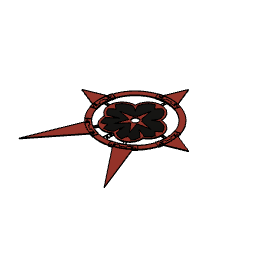
ワカモ_ヘイロー_mk1 v11 (Autodesk Fusion 360 design; units mm, degrees)
Autodesk Fusion 360 part; units mm, degrees
sketch "スケッチ1" plane through (0, 0, 0) normal (0, 0, 1) x (1, 0, 0) in component "main"
  circle A0 centre (0, 0) radius 95
  circle A1 centre (0, 0) radius 10
  line L0 (0, 0) -> (0, 47.5) construction
  line L1 (0, 0) -> (47.5, 0) construction
  line L2 (0, 0) -> (-47.5, 0) construction
  line L3 (0, 0) -> (23.75, -41.1362) construction
  line L4 (0, 0) -> (-23.75, -41.1362) construction
  line L5 (0, 47.5) -> (-6.6163, 13.462)
  line L6 (0, 47.5) -> (6.6163, 13.462)
  line L7 (-47.5, 0) -> (-13.462, 6.6163)
  line L8 (-47.5, 0) -> (-13.462, -6.6163)
  line L9 (-23.75, -41.1362) -> (-12.4609, -8.3502)
  line L10 (-23.75, -41.1362) -> (-1.0011, -14.9666)
  line L11 (23.75, -41.1362) -> (1.0011, -14.9666)
  line L12 (23.75, -41.1362) -> (12.4609, -8.3502)
  line L13 (47.5, 0) -> (13.462, -6.6163)
  line L14 (47.5, 0) -> (13.462, 6.6163)
  arc A2 (-13.462, -6.6163) -> (-12.4609, -8.3502) centre (0, 0) ccw
  arc A3 (-1.0011, -14.9666) -> (1.0011, -14.9666) centre (0, 0) ccw
  arc A4 (12.4609, -8.3502) -> (13.462, -6.6163) centre (0, 0) ccw
  arc A5 (13.462, 6.6163) -> (6.6163, 13.462) centre (0, 0) ccw
  arc A6 (-6.6163, 13.462) -> (-13.462, 6.6163) centre (0, 0) ccw
  circle A7 centre (0, 40) radius 40 construction
  circle A8 centre (40, 0) radius 40 construction
  circle A9 centre (-40, 0) radius 40 construction
  circle A10 centre (-23.75, -41.1362) radius 35 construction
  circle A11 centre (23.75, -41.1362) radius 35 construction
  arc A12 (40, 40) -> (-40, 40) centre (0, 40) ccw
  arc A13 (58.304, -35.5663) -> (40, 40) centre (40, 0) ccw
  arc A14 (-40, 40) -> (-58.304, -35.5663) centre (-40, 0) ccw
  arc A15 (0, -66.8449) -> (58.304, -35.5663) centre (23.75, -41.1362) ccw
  arc A16 (-58.304, -35.5663) -> (0, -66.8449) centre (-23.75, -41.1362) ccw
  circle A17 centre (0, 40) radius 34 construction
  circle A18 centre (-40, 0) radius 34 construction
  circle A19 centre (40, 0) radius 34 construction
  circle A20 centre (-23.75, -41.1362) radius 29 construction
  circle A21 centre (23.75, -41.1362) radius 29 construction
  line L15 (0, 40) -> (0, 59.4286) construction
  line L16 (0, 59.4286) -> (-10.7604, 72.2523)
  line L17 (0, 59.4286) -> (10.7604, 72.2523)
  line L18 (-40, 0) -> (-59.4286, 0) construction
  line L19 (-59.4286, 0) -> (-72.2523, 10.7604)
  line L20 (-59.4286, 0) -> (-72.2523, -10.7604)
  line L21 (40, 0) -> (59.4286, 0) construction
  line L22 (59.4286, 0) -> (72.2523, 10.7604)
  line L23 (59.4286, 0) -> (72.2523, -10.7604)
  line L24 (-23.75, -41.1362) -> (-31, -53.6936) construction
  line L25 (-31, -53.6936) -> (-28.1602, -69.7989)
  line L26 (-31, -53.6936) -> (-46.3675, -59.2869)
  line L27 (23.75, -41.1362) -> (31, -53.6936) construction
  line L28 (31, -53.6936) -> (28.1602, -69.7989)
  line L29 (31, -53.6936) -> (46.3675, -59.2869)
  arc A22 (33.997, 39.547) -> (10.7604, 72.2523) centre (0, 40) ccw
  arc A23 (-10.7604, 72.2523) -> (-33.997, 39.547) centre (0, 40) ccw
  arc A24 (-39.547, 33.997) -> (-72.2523, 10.7604) centre (-40, 0) ccw
  arc A25 (-72.2523, -10.7604) -> (-56.7833, -29.5689) centre (-40, 0) ccw
  arc A26 (-52.5768, -37.9714) -> (-46.3675, -59.2869) centre (-23.75, -41.1362) ccw
  arc A27 (-28.1602, -69.7989) -> (-4.0421, -62.4106) centre (-23.75, -41.1362) ccw
  arc A28 (4.0421, -62.4106) -> (28.1602, -69.7989) centre (23.75, -41.1362) ccw
  arc A29 (46.3675, -59.2869) -> (52.5768, -37.9714) centre (23.75, -41.1362) ccw
  arc A30 (56.7833, -29.5689) -> (72.2523, -10.7604) centre (40, 0) ccw
  arc A31 (72.2523, 10.7604) -> (39.547, 33.997) centre (40, 0) ccw
  line L30 (0, 0) -> (-33.3417, 33.3417) construction
  circle A32 centre (0, 0) radius 35 construction
  line L31 (-39.547, 33.997) -> (-24.7487, 24.7487)
  line L32 (-33.997, 39.547) -> (-24.7487, 24.7487)
  line L33 (0, 0) -> (33.3417, 33.3417) construction
  line L34 (33.997, 39.547) -> (24.7487, 24.7487)
  line L35 (39.547, 33.997) -> (24.7487, 24.7487)
  line L36 (0, 0) -> (-51.296, -32.0687) construction
  line L37 (-56.7833, -29.5689) -> (-29.6777, -18.5536)
  line L38 (-29.6777, -18.5536) -> (-52.5768, -37.9714)
  line L39 (0, 0) -> (0, -57.7776) construction
  line L40 (-4.0421, -62.4106) -> (0, -35)
  line L41 (0, -35) -> (4.0421, -62.4106)
  line L42 (0, 0) -> (51.296, -32.0687) construction
  line L43 (52.5768, -37.9714) -> (29.6777, -18.5536)
  line L44 (56.7833, -29.5689) -> (29.6777, -18.5536)
  line L45 (-2.5, 79.9218) -> (-2.5, 94.9671)
  line L46 (2.5, 79.9218) -> (2.5, 94.9671)
  line L47 (-94.9671, 2.5) -> (-79.9218, 2.5)
  line L48 (-94.9671, -2.5) -> (-79.9218, -2.5)
  line L49 (79.9218, 2.5) -> (94.9671, 2.5)
  line L50 (79.9218, -2.5) -> (94.9671, -2.5)
  line L51 (38.5875, -72.8355) -> (44.8782, -83.7314)
  line L52 (43.7837, -69.8355) -> (50.0744, -80.7314)
  line L53 (-43.7837, -69.8355) -> (-50.0744, -80.7314)
  line L54 (-38.5875, -72.8355) -> (-44.8782, -83.7314)
  circle A33 centre (-42.75, -74.0452) radius 1.6
  circle A34 centre (42.75, -74.0452) radius 1.6
  line L55 (-73.3227, -81.9987) -> (-34.3516, -104.4987) construction
  line L56 (-53.8371, -93.2487) -> (-31, -53.6936) construction
  line L57 (-71.3227, -78.5346) -> (-70.094, -77.6742)
  line L58 (-70.094, -77.6742) -> (-69.094, -75.9421)
  line L59 (-69.094, -75.9421) -> (-68.9632, -74.4479)
  line L60 (-73.3227, -81.9987) -> (-71.3227, -78.5346)
  line L61 (-68.9632, -74.4479) -> (-68.2035, -73.1319)
  line L62 (-56.7679, -82.325) -> (-58.7679, -85.7891)
  arc A35 (-68.2035, -73.1319) -> (-56.7679, -82.325) centre (0, 0) ccw
  line L63 (-58.7679, -85.7891) -> (-51.8397, -89.7891)
  arc A36 (-42.9115, -90.325) -> (-29.2324, -95.6319) centre (0, 0) ccw
  line L64 (-29.9921, -96.9479) -> (-29.2324, -95.6319)
  line L65 (-31.2208, -97.8082) -> (-29.9921, -96.9479)
  line L66 (-32.2208, -99.5403) -> (-31.2208, -97.8082)
  line L67 (-32.3516, -101.0346) -> (-32.2208, -99.5403)
  line L68 (-34.3516, -104.4987) -> (-32.3516, -101.0346)
  line L69 (-42.9115, -90.325) -> (-44.9115, -93.7891)
  line L70 (-44.9115, -93.7891) -> (-51.8397, -89.7891)
  line L71 (-69.594, -76.8082) -> (-73.9241, -74.3082) construction
  circle A37 centre (-73.9241, -74.3082) radius 1.5
  circle A38 centre (-27.3907, -101.1742) radius 1.5
  circle A39 centre (27.3907, -101.1742) radius 1.5
  line L72 (31.2208, -97.8082) -> (29.9921, -96.9479)
  line L73 (29.9921, -96.9479) -> (29.2324, -95.6319)
  arc A40 (29.2324, -95.6319) -> (42.9115, -90.325) centre (0, 0) ccw
  line L74 (32.2208, -99.5403) -> (31.2208, -97.8082)
  line L75 (32.3516, -101.0346) -> (32.2208, -99.5403)
  line L76 (34.3516, -104.4987) -> (32.3516, -101.0346)
  line L77 (42.9115, -90.325) -> (44.9115, -93.7891)
  line L78 (44.9115, -93.7891) -> (51.8397, -89.7891)
  line L79 (58.7679, -85.7891) -> (51.8397, -89.7891)
  line L80 (56.7679, -82.325) -> (58.7679, -85.7891)
  arc A41 (56.7679, -82.325) -> (68.2035, -73.1319) centre (0, 0) ccw
  line L81 (68.9632, -74.4479) -> (68.2035, -73.1319)
  line L82 (69.094, -75.9421) -> (68.9632, -74.4479)
  line L83 (70.094, -77.6742) -> (69.094, -75.9421)
  line L84 (71.3227, -78.5346) -> (70.094, -77.6742)
  line L85 (73.3227, -81.9987) -> (71.3227, -78.5346)
  circle A42 centre (73.9241, -74.3082) radius 1.5
  circle A43 centre (101.3148, -26.8661) radius 1.5
  line L86 (100.3148, -21.8661) -> (98.9554, -22.5)
  line L87 (98.9554, -22.5) -> (97.4359, -22.5)
  arc A44 (97.4359, -22.5) -> (99.6795, -8) centre (0, 0) ccw
  line L88 (102.3148, -21.8661) -> (100.3148, -21.8661)
  line L89 (103.6743, -22.5) -> (102.3148, -21.8661)
  line L90 (107.6743, -22.5) -> (103.6743, -22.5)
  line L91 (99.6795, -8) -> (103.6795, -8)
  line L92 (103.6795, -8) -> (103.6795, 0)
  line L93 (103.6795, 8) -> (103.6795, 0)
  line L94 (99.6795, 8) -> (103.6795, 8)
  arc A45 (99.6795, 8) -> (97.4359, 22.5) centre (0, 0) ccw
  line L95 (98.9554, 22.5) -> (97.4359, 22.5)
  line L96 (100.3148, 21.8661) -> (98.9554, 22.5)
  line L97 (102.3148, 21.8661) -> (100.3148, 21.8661)
  line L98 (103.6743, 22.5) -> (102.3148, 21.8661)
  line L99 (107.6743, 22.5) -> (103.6743, 22.5)
  circle A46 centre (101.3148, 26.8661) radius 1.5
  circle A47 centre (26.8661, 101.3148) radius 1.5
  line L100 (21.8661, 100.3148) -> (22.5, 98.9554)
  line L101 (22.5, 98.9554) -> (22.5, 97.4359)
  arc A48 (22.5, 97.4359) -> (8, 99.6795) centre (0, 0) ccw
  line L102 (21.8661, 102.3148) -> (21.8661, 100.3148)
  line L103 (22.5, 103.6743) -> (21.8661, 102.3148)
  line L104 (22.5, 107.6743) -> (22.5, 103.6743)
  line L105 (8, 99.6795) -> (8, 103.6795)
  line L106 (8, 103.6795) -> (0, 103.6795)
  line L107 (-8, 103.6795) -> (0, 103.6795)
  line L108 (-8, 99.6795) -> (-8, 103.6795)
  arc A49 (-8, 99.6795) -> (-22.5, 97.4359) centre (0, 0) ccw
  line L109 (-22.5, 98.9554) -> (-22.5, 97.4359)
  line L110 (-21.8661, 100.3148) -> (-22.5, 98.9554)
  line L111 (-21.8661, 102.3148) -> (-21.8661, 100.3148)
  line L112 (-22.5, 103.6743) -> (-21.8661, 102.3148)
  line L113 (-22.5, 107.6743) -> (-22.5, 103.6743)
  circle A50 centre (-26.8661, 101.3148) radius 1.5
  circle A51 centre (-101.3148, 26.8661) radius 1.5
  line L114 (-100.3148, 21.8661) -> (-98.9554, 22.5)
  line L115 (-98.9554, 22.5) -> (-97.4359, 22.5)
  arc A52 (-97.4359, 22.5) -> (-99.6795, 8) centre (0, 0) ccw
  line L116 (-102.3148, 21.8661) -> (-100.3148, 21.8661)
  line L117 (-103.6743, 22.5) -> (-102.3148, 21.8661)
  line L118 (-107.6743, 22.5) -> (-103.6743, 22.5)
  line L119 (-99.6795, 8) -> (-103.6795, 8)
  line L120 (-103.6795, 8) -> (-103.6795, 0)
  line L121 (-103.6795, -8) -> (-103.6795, 0)
  line L122 (-99.6795, -8) -> (-103.6795, -8)
  arc A53 (-99.6795, -8) -> (-97.4359, -22.5) centre (0, 0) ccw
  line L123 (-98.9554, -22.5) -> (-97.4359, -22.5)
  line L124 (-100.3148, -21.8661) -> (-98.9554, -22.5)
  line L125 (-102.3148, -21.8661) -> (-100.3148, -21.8661)
  line L126 (-103.6743, -22.5) -> (-102.3148, -21.8661)
  line L127 (-107.6743, -22.5) -> (-103.6743, -22.5)
  circle A54 centre (-101.3148, -26.8661) radius 1.5
  arc A55 (-107.6743, -22.5) -> (-73.3227, -81.9987) centre (0, 0) ccw
  arc A56 (-22.5, 107.6743) -> (-107.6743, 22.5) centre (0, 0) ccw
  arc A57 (107.6743, 22.5) -> (22.5, 107.6743) centre (0, 0) ccw
  arc A58 (-34.3516, -104.4987) -> (34.3516, -104.4987) centre (0, 0) ccw
  arc A59 (73.3227, -81.9987) -> (107.6743, -22.5) centre (0, 0) ccw
  line L128 (-5, -70.6902) -> (-5, -94.8683)
  line L129 (5, -70.6902) -> (5, -94.8683)
  circle A60 centre (0, -75) radius 2.6
  circle A61 centre (0, -87) radius 2.6
  dimension "d1" = 220
  dimension "d2" = 190
  dimension "d3" = 20
  dimension "d4" = 47.5
  dimension "d5" = 47.5
  dimension "d6" = 47.5
  dimension "d7" = 60
  dimension "d8" = 47.5
  dimension "d9" = 60
  dimension "d10" = 47.5
  dimension "d11" = 30
  dimension "d12" = 11
  dimension "d13" = 11
  dimension "d14" = 11
  dimension "d15" = 11
  dimension "d16" = 11
  dimension "d17" = 11
  dimension "d18" = 11
  dimension "d19" = 11
  dimension "d20" = 11
  dimension "d21" = 11
  dimension "d22" = 40
  dimension "d23" = 40
  dimension "d24" = 40
  dimension "d25" = 80
  dimension "d26" = 80
  dimension "d27" = 80
  dimension "d28" = 70
  dimension "d29" = 70
  dimension "d30" = 68
  dimension "d31" = 68
  dimension "d32" = 68
  dimension "d33" = 58
  dimension "d34" = 58
  dimension "d35" = 19.4286
  dimension "d36" = 140
  dimension "d37" = 140
  dimension "d38" = 19.4286
  dimension "d39" = 140
  dimension "d40" = 140
  dimension "d41" = 19.4286
  dimension "d42" = 140
  dimension "d43" = 140
  dimension "d44" = 14.5
  dimension "d45" = 140
  dimension "d46" = 140
  dimension "d47" = 14.5
  dimension "d48" = 140
  dimension "d49" = 140
  dimension "d50" = 70
  dimension "d52" = 5
  dimension "d53" = 5
  dimension "d54" = 6
  dimension "d55" = 6
  dimension "d56" = 5
  dimension "d67" = 3.2
  dimension "d68" = 38
  dimension "d69" = 3
  dimension "d70" = 3.2
  dimension "d71" = 38
  dimension "d72" = 3
  dimension "d73" = 45
  dimension "d75" = 25
  dimension "d76" = 1.5
  dimension "d77" = 2
  dimension "d78" = 25
  dimension "d79" = 1.5
  dimension "d80" = 4
  dimension "d83" = 100
  dimension "d84" = 4
  dimension "d85" = 8
  dimension "d86" = 5
  dimension "d87" = 3
  dimension "d89" = 360
  dimension "d111" = 10
  dimension "d112" = 5.2
  dimension "d113" = 5.2
  dimension "d114" = 12
  dimension "d115" = 87
  constraint coincident A0.centre A1.centre
  constraint concentric A0 A58
  constraint concentric A0 A1
  constraint vertical L0
  constraint perpendicular L0 L1
  constraint perpendicular L0 L2
  constraint concentric A0 A2
  constraint coincident L5.end A2
  constraint coincident L6.end A2
  constraint coincident L10.end A2
  constraint coincident L11.end A2
  constraint coincident L12.end A2
  constraint coincident L13.end A2
  constraint coincident L14.end A2
  constraint concentric A2 A3
  constraint concentric A3 A4
  constraint concentric A4 A5
  constraint concentric A5 A6
  constraint coincident L0 A7.centre
  constraint coincident L1 A8.centre
  constraint coincident L2 A9.centre
  constraint coincident L4.end L9.start
  constraint coincident L3.end L11.start
  constraint coincident A7 A12.start
  constraint coincident A8 A12.start
  constraint coincident A9 A12.end
  constraint coincident A7 A12.end
  constraint coincident A7.centre A12.centre
  constraint coincident A11 A13.start
  constraint coincident A8.centre A13.centre
  constraint coincident A10 A14.end
  constraint coincident A9.centre A14.centre
  constraint coincident A13.start A15.end
  constraint coincident A10 A15.start
  constraint coincident A14.end A16.start
  constraint coincident A11 A15.start
  constraint concentric A7 A17
  constraint concentric A14 A18
  constraint concentric A8 A19
  constraint concentric A10 A20
  constraint concentric A11 A21
  constraint parallel L0 L15
  constraint coincident A17 L16.end
  constraint coincident A17 L17.end
  constraint parallel L2 L18
  constraint coincident A18 L19.end
  constraint coincident A18 L20.end
  constraint parallel L1 L21
  constraint coincident A19 L22.end
  constraint coincident A19 L23.end
  constraint parallel L4 L24
  constraint coincident A20 L25.end
  constraint coincident A20 L26.end
  constraint coincident A21 L28.end
  constraint coincident A21 L29.end
  constraint coincident L17.end A22.end
  constraint coincident A8 A22.start
  constraint coincident L16.end A23.start
  constraint coincident A9 A23.end
  constraint coincident L19.end A24.end
  constraint coincident A7 A24.start
  constraint coincident L20.end A25.start
  constraint coincident A10 A25.end
  constraint coincident L26.end A26.end
  constraint coincident A9 A26.start
  constraint coincident L25.end A27.start
  constraint coincident A11 A27.end
  constraint coincident L28.end A28.end
  constraint coincident A10 A28.start
  constraint coincident L29.end A29.start
  constraint coincident A8 A29.end
  constraint coincident L23.end A30.end
  constraint coincident A11 A30.start
  constraint coincident L22.end A31.start
  constraint coincident A7 A31.end
  constraint coincident A17 L30.end
  constraint coincident A18 L30.end
  constraint concentric A6 A32
  constraint coincident A32 L31.end
  constraint coincident L30 L31.end
  constraint coincident A17 L33.end
  constraint coincident A19 L33.end
  constraint coincident L33 L34.end
  constraint coincident A32 L34.end
  constraint coincident A20 L36.end
  constraint coincident A18 L36.end
  constraint coincident L36 L37.end
  constraint coincident A32 L37.end
  constraint coincident A20 L39.end
  constraint coincident A21 L39.end
  constraint coincident L39 L40.end
  constraint coincident A32 L40.end
  constraint coincident A21 L42.end
  constraint coincident A19 L42.end
  constraint coincident L42 L43.end
  constraint coincident A32 L43.end
  constraint coincident A12 L45.start
  constraint coincident A0 L45.end
  constraint vertical L45
  constraint coincident A7 L46.start
  constraint coincident A0 L46.end
  constraint parallel L45 L46
  constraint symmetric L15 L45 L46
  constraint parallel L3 L27
  constraint coincident A0 L47.start
  constraint coincident A9 L47.end
  constraint coincident A0 L48.start
  constraint coincident A14 L48.end
  constraint coincident A13 L49.start
  constraint coincident A0 L49.end
  constraint parallel L48 L49
  constraint coincident A13 L50.start
  constraint coincident A0 L50.end
  constraint parallel L49 L50
  constraint coincident A15 L51.start
  constraint coincident A0 L51.end
  constraint coincident A15 L52.start
  constraint coincident A0 L52.end
  constraint parallel L51 L52
  constraint coincident A10 L53.start
  constraint coincident A0 L53.end
  constraint coincident A16 L54.start
  constraint coincident A0 L54.end
  constraint symmetric L18 L47 L48
  constraint symmetric L24 L53 L54
  constraint symmetric L27 L51 L52
  constraint symmetric L21 L49 L50
  constraint parallel L24 L53
  constraint perpendicular L24 L55
  constraint midpoint L55 L56.start
  constraint perpendicular L55 L60
  constraint coincident L59.end L60
  constraint collinear L60 L61
  constraint parallel L53 L62
  constraint coincident L56 L63.end
  constraint perpendicular L56 L63
  constraint symmetric L55.start L56 L55.end
  constraint symmetric L56 L57.start L67.start
  constraint symmetric L56 L57.end L66.start
  constraint symmetric L56 L58.end L65.start
  constraint symmetric L56 L59.end L64.start
  constraint symmetric L56 L62.end L69.end
  constraint symmetric L56 L61.end A36.end
  constraint symmetric L56 A35 A36
  constraint symmetric L56 L62.start A36.start
  constraint symmetric L56 L63.end L70.end
  constraint coincident L55 L68.start
  constraint midpoint L58 L71.start
  constraint perpendicular L58 L71
  constraint coincident L71.end A37.centre
  constraint symmetric L56 A37 A38
  constraint concentric A55 A58
  constraint concentric A56 A58
  constraint concentric A57 A58
  constraint concentric A58 A59
  constraint coincident A10 L128.start
  constraint coincident A0 L128.end
  constraint vertical L128
  constraint coincident A11 L129.start
  constraint coincident A0 L129.end
  constraint parallel L128 L129
  constraint symmetric L39 L128 L129
  measures "d1" diameter of A58
  measures "d2" diameter of A0
  measures "d3" diameter of A1
  measures "d4" distance of A0.centre L0.end
  measures "d5" distance of A0.centre L1.end
  measures "d6" distance of A0.centre L2.end
  measures "d7" angle of L1 L3
  measures "d8" distance of A0.centre L3.end
  measures "d9" angle of L2 L4
  measures "d10" distance of A0.centre L4.end
  measures "d11" diameter of A2
  measures "d12" angle of L0 L5
  measures "d13" angle of L0 L6
  measures "d14" angle of L1 L14
  measures "d15" angle of L1 L13
  measures "d16" angle of L3 L12
  measures "d17" angle of L3 L11
  measures "d18" angle of L2 L7
  measures "d19" angle of L2 L8
  measures "d20" angle of L4 L9
  measures "d21" angle of L4 L10
  measures "d22" distance of A0.centre A7.centre
  measures "d23" distance of A0.centre A8.centre
  measures "d24" distance of A0.centre A9.centre
  measures "d25" diameter of A7
  measures "d26" diameter of A8
  measures "d27" diameter of A9
  measures "d28" diameter of A10
  measures "d29" diameter of A11
  measures "d30" diameter of A17
  measures "d31" diameter of A18
  measures "d32" diameter of A19
  measures "d33" diameter of A20
  measures "d34" diameter of A21
  measures "d35" distance of A7.centre L15.end
  measures "d36" angle of L15 L16
  measures "d37" angle of L15 L17
  measures "d38" distance of A9.centre L18.end
  measures "d39" angle of L18 L20
  measures "d40" angle of L18 L19
  measures "d41" distance of A8.centre L21.end
  measures "d42" angle of L21 L22
  measures "d43" angle of L21 L23
  measures "d44" distance of L4.end L24.end
  measures "d45" angle of L24 L26
  measures "d46" angle of L24 L25
  measures "d47" distance of L3.end L27.end
  measures "d48" angle of L27 L28
  measures "d49" angle of L27 L29
  measures "d50" diameter of A32
  measures "d52" distance of L45 L46
  measures "d53" distance of L47 L48
  measures "d54" distance of L53 L54
  measures "d55" distance of L51 L52
  measures "d56" distance of L49 L50
  measures "d67" diameter of A33
  measures "d68" distance of L4.end A33.centre
  measures "d69" distance of L54 A33.centre
  measures "d70" diameter of A34
  measures "d71" distance of L3.end A34.centre
  measures "d72" distance of L51 A34.centre
  measures "d73" distance of L55.start L55.end
  measures "d75" angle of L57 L60
  measures "d76" distance of L57.start L57.end
  measures "d77" distance of L57.end L58.end
  measures "d78" angle of L59 L60
  measures "d79" distance of L58.end L59.end
  measures "d80" distance of L55 L57.start
  measures "d83" radius of A35
  measures "d84" distance of L62.end L62.start
  measures "d85" distance of L62.end L63.end
  measures "d86" distance of L71.start L71.end
  measures "d87" diameter of A37
  measures "d111" distance of L128 L129
  measures "d112" diameter of A60
  measures "d113" diameter of A61
  measures "d114" distance of A60.centre A61.centre
  measures "d115" distance of A0.centre A61.centre
extrude "押し出し1" add sketch "スケッチ1" along normal blind 2 contours L57 L58 L59 L60 L61 L62 A35 L63 A36 L64 L65 L66 L67 L68 L69 L70 L72 L73 A40 L74 L75 L76 L77 L78 L79 L80 A41 L81 L82 L83 L84 L85 L86 L87 A44 L88 L89 L90 L91 L92 L93 L94 A45 L95 L96 L97 L98 L99 L100 L101 A48 L102 L103 L104 L105 L106 L107 L108 A49 L109 L110 L111 L112 L113 L114 L115 A52 L116 L117 L118 L119 L120 L121 L122 A53 L123 L124 L125 L126 L127 A55 A56 A57 A58 A59 makes body 1 in component "main"
extrude "押し出し2" add sketch "スケッチ1" along normal blind 2 separate body contours A0 A13 L49 L50 | A0 A12 L45 L46 | A0 A15 L51 L52 | A0 A14 L47 L48 | A0 A15 A16 L128 L129 | A0 A16 L53 L54 | A33 | A34 makes body 2 at (-45.3226, -73.8337, 0) makes body 3 at (-84.9601, -1.9446, 0) makes body 4 at (45.3226, -73.8337, 0) makes body 5 at (-1.9446, 84.9601, 0) makes body 6 at (84.9601, 1.9446, 2) makes body 7 at (-0.0648, -93.1878, 0) in component "main"
extrude "押し出し3" add sketch "スケッチ1" along normal blind 2 separate body contours A12 A13 A14 A15 A16 makes body 8 in component "main"
extrude "押し出し4" add sketch "スケッチ1" along normal blind 2 separate body contours L16 L17 L19 L20 L22 L23 L25 L26 L28 L29 A22 A23 A24 A25 A26 A27 A28 A29 A30 A31 L31 L32 L34 L35 L37 L38 L40 L41 L43 L44 makes body 9 in component "main"
extrude "押し出し5" add sketch "スケッチ1" along normal blind 2 separate body contours L5 L6 L7 L8 L9 L10 L11 L12 L13 L14 A2 A3 A4 A5 A6 makes body 10 in component "main"
sketch "スケッチ1 (2)" plane through (0, 0, 2) normal (0, 0, 1) x (-1, 0, 0) in component "突起a"
  circle A0 centre (-73.9241, 74.3082) radius 1.5
  circle A1 centre (101.3148, 26.8661) radius 1.5
  circle A2 centre (-27.3907, 101.1742) radius 1.5
  circle A3 centre (-26.8661, -101.3148) radius 1.5
  circle A4 centre (27.3907, 101.1742) radius 1.5
  circle A5 centre (101.3148, -26.8661) radius 1.5
  circle A6 centre (-101.3148, 26.8661) radius 1.5
  circle A7 centre (-101.3148, -26.8661) radius 1.5
  circle A8 centre (26.8661, -101.3148) radius 1.5
  circle A9 centre (73.9241, 74.3082) radius 1.5
  circle A10 centre (0, 0) radius 95
  line L0 (-71.3227, 78.5346) -> (-73.3227, 81.9987)
  arc A11 (-73.3227, 81.9987) -> (-107.6743, 22.5) centre (0, 0) ccw
  line L1 (-107.6743, 22.5) -> (-103.6743, 22.5)
  line L2 (-103.6743, 22.5) -> (-102.3148, 21.8661)
  line L3 (-102.3148, 21.8661) -> (-100.3148, 21.8661)
  line L4 (-100.3148, 21.8661) -> (-98.9554, 22.5)
  line L5 (-98.9554, 22.5) -> (-97.4359, 22.5)
  arc A12 (-97.4359, 22.5) -> (-99.6795, 8) centre (0, 0) ccw
  line L6 (-99.6795, 8) -> (-103.6795, 8)
  line L7 (-103.6795, 8) -> (-103.6795, -8)
  line L8 (-103.6795, -8) -> (-99.6795, -8)
  arc A13 (-99.6795, -8) -> (-97.4359, -22.5) centre (0, 0) ccw
  line L9 (-97.4359, -22.5) -> (-98.9554, -22.5)
  line L10 (-98.9554, -22.5) -> (-100.3148, -21.8661)
  line L11 (-100.3148, -21.8661) -> (-102.3148, -21.8661)
  line L12 (-102.3148, -21.8661) -> (-103.6743, -22.5)
  line L13 (-103.6743, -22.5) -> (-107.6743, -22.5)
  arc A14 (-107.6743, -22.5) -> (-22.5, -107.6743) centre (0, 0) ccw
  line L14 (-22.5, -107.6743) -> (-22.5, -103.6743)
  line L15 (-22.5, -103.6743) -> (-21.8661, -102.3148)
  line L16 (-21.8661, -102.3148) -> (-21.8661, -100.3148)
  line L17 (-21.8661, -100.3148) -> (-22.5, -98.9554)
  line L18 (-22.5, -98.9554) -> (-22.5, -97.4359)
  arc A15 (-22.5, -97.4359) -> (-8, -99.6795) centre (0, 0) ccw
  line L19 (-8, -99.6795) -> (-8, -103.6795)
  line L20 (-8, -103.6795) -> (8, -103.6795)
  line L21 (8, -103.6795) -> (8, -99.6795)
  arc A16 (8, -99.6795) -> (22.5, -97.4359) centre (0, 0) ccw
  line L22 (22.5, -97.4359) -> (22.5, -98.9554)
  line L23 (22.5, -98.9554) -> (21.8661, -100.3148)
  line L24 (21.8661, -100.3148) -> (21.8661, -102.3148)
  line L25 (21.8661, -102.3148) -> (22.5, -103.6743)
  line L26 (22.5, -103.6743) -> (22.5, -107.6743)
  arc A17 (22.5, -107.6743) -> (107.6743, -22.5) centre (0, 0) ccw
  line L27 (107.6743, -22.5) -> (103.6743, -22.5)
  line L28 (103.6743, -22.5) -> (102.3148, -21.8661)
  line L29 (102.3148, -21.8661) -> (100.3148, -21.8661)
  line L30 (100.3148, -21.8661) -> (98.9554, -22.5)
  line L31 (98.9554, -22.5) -> (97.4359, -22.5)
  arc A18 (97.4359, -22.5) -> (99.6795, -8) centre (0, 0) ccw
  line L32 (99.6795, -8) -> (103.6795, -8)
  line L33 (103.6795, -8) -> (103.6795, 8)
  line L34 (103.6795, 8) -> (99.6795, 8)
  arc A19 (99.6795, 8) -> (97.4359, 22.5) centre (0, 0) ccw
  line L35 (97.4359, 22.5) -> (98.9554, 22.5)
  line L36 (98.9554, 22.5) -> (100.3148, 21.8661)
  line L37 (100.3148, 21.8661) -> (102.3148, 21.8661)
  line L38 (102.3148, 21.8661) -> (103.6743, 22.5)
  line L39 (103.6743, 22.5) -> (107.6743, 22.5)
  arc A20 (107.6743, 22.5) -> (73.3227, 81.9987) centre (0, 0) ccw
  line L40 (73.3227, 81.9987) -> (71.3227, 78.5346)
  line L41 (71.3227, 78.5346) -> (70.094, 77.6742)
  line L42 (70.094, 77.6742) -> (69.094, 75.9421)
  line L43 (69.094, 75.9421) -> (68.9632, 74.4479)
  line L44 (68.9632, 74.4479) -> (68.2035, 73.1319)
  arc A21 (68.2035, 73.1319) -> (56.7679, 82.325) centre (0, 0) ccw
  line L45 (56.7679, 82.325) -> (58.7679, 85.7891)
  line L46 (58.7679, 85.7891) -> (44.9115, 93.7891)
  line L47 (44.9115, 93.7891) -> (42.9115, 90.325)
  arc A22 (42.9115, 90.325) -> (29.2324, 95.6319) centre (0, 0) ccw
  line L48 (29.2324, 95.6319) -> (29.9921, 96.9479)
  line L49 (29.9921, 96.9479) -> (31.2208, 97.8082)
  line L50 (31.2208, 97.8082) -> (32.2208, 99.5403)
  line L51 (32.2208, 99.5403) -> (32.3516, 101.0346)
  line L52 (32.3516, 101.0346) -> (34.3516, 104.4987)
  arc A23 (34.3516, 104.4987) -> (-34.3516, 104.4987) centre (0, 0) ccw
  line L53 (-34.3516, 104.4987) -> (-32.3516, 101.0346)
  line L54 (-32.3516, 101.0346) -> (-32.2208, 99.5403)
  line L55 (-32.2208, 99.5403) -> (-31.2208, 97.8082)
  line L56 (-31.2208, 97.8082) -> (-29.9921, 96.9479)
  line L57 (-29.9921, 96.9479) -> (-29.2324, 95.6319)
  arc A24 (-29.2324, 95.6319) -> (-42.9115, 90.325) centre (0, 0) ccw
  line L58 (-42.9115, 90.325) -> (-44.9115, 93.7891)
  line L59 (-44.9115, 93.7891) -> (-58.7679, 85.7891)
  line L60 (-58.7679, 85.7891) -> (-56.7679, 82.325)
  arc A25 (-56.7679, 82.325) -> (-68.2035, 73.1319) centre (0, 0) ccw
  line L61 (-68.2035, 73.1319) -> (-68.9632, 74.4479)
  line L62 (-68.9632, 74.4479) -> (-69.094, 75.9421)
  line L63 (-69.094, 75.9421) -> (-70.094, 77.6742)
  line L64 (-70.094, 77.6742) -> (-71.3227, 78.5346)
  line L65 (73.3227, 81.9987) -> (71.3227, 78.5346)
  line L66 (70.094, 77.6742) -> (71.3227, 78.5346)
  line L67 (70.094, 77.6742) -> (69.094, 75.9421)
  line L68 (69.094, 75.9421) -> (68.9632, 74.4479)
  line L69 (68.9632, 74.4479) -> (68.2035, 73.1319)
  line L70 (42.9115, 90.325) -> (44.9115, 93.7891)
  line L71 (44.9115, 93.7891) -> (58.7679, 85.7891)
  line L72 (58.7679, 85.7891) -> (56.7679, 82.325)
  line L73 (29.2324, 95.6319) -> (29.9921, 96.9479)
  line L74 (29.9921, 96.9479) -> (31.2208, 97.8082)
  line L75 (31.2208, 97.8082) -> (32.2208, 99.5403)
  line L76 (32.2208, 99.5403) -> (32.3516, 101.0346)
  line L77 (32.3516, 101.0346) -> (34.3516, 104.4987)
  line L78 (51.8397, 89.7891) -> (130.3397, 225.7551) construction
  line L79 (73.3227, 81.9987) -> (130.3397, 225.7551)
  line L80 (130.3397, 225.7551) -> (34.3516, 104.4987)
  line L81 (66.2079, 74.9434) -> (70.5417, 82.4496)
  line L82 (70.5417, 82.4496) -> (68.8096, 83.4496)
  line L83 (68.8096, 83.4496) -> (64.668, 76.2761)
  line L84 (73.3227, 81.9987) -> (34.3516, 104.4987)
  arc A26 (68.2035, 73.1319) -> (66.2079, 74.9434) centre (0, 0) ccw
  arc A27 (64.668, 76.2761) -> (56.7679, 82.325) centre (0, 0) ccw
  line L85 (31.7989, 94.8094) -> (36.1326, 102.3157)
  line L86 (37.8647, 101.3157) -> (33.7231, 94.1422)
  line L87 (36.1326, 102.3157) -> (37.8647, 101.3157)
  arc A28 (42.9115, 90.325) -> (33.7231, 94.1422) centre (0, 0) ccw
  arc A29 (31.7989, 94.8094) -> (29.2324, 95.6319) centre (0, 0) ccw
  dimension "d90" = 157
  dimension "d91" = 1
  dimension "d92" = 2
  dimension "d93" = 2
  constraint coincident A20.end L40.start
  constraint coincident L40.end L41.start
  constraint coincident L41.end L42.start
  constraint coincident L42.end L43.start
  constraint coincident L43.end L44.start
  constraint coincident L44.end A21.start
  constraint coincident A21.end L45.start
  constraint coincident A22.end L48.start
  constraint coincident L47.end A22.start
  constraint coincident A10.centre A11.centre
  constraint parallel L47 L70
  constraint coincident L45.end L46.start
  constraint perpendicular L45 L71
  constraint coincident L48.end L49.start
  constraint parallel L49 L74
  constraint coincident L50.end L51.start
  constraint parallel L50 L75
  constraint coincident L51.end L52.start
  constraint coincident L52.end A23.start
  constraint midpoint L71 L78.start
  constraint perpendicular L71 L78
  constraint parallel L78 L81
  constraint perpendicular L81 L82
  constraint coincident L83.end A26
  constraint perpendicular L82 L83
  constraint concentric A26 A27
  constraint symmetric L78 L81.start L85.start
  constraint symmetric L78 L81.end L85.end
  constraint symmetric L78 L82.end L86.start
  constraint symmetric L78 L83.end L86.end
  constraint concentric A28 A29
  measures "d90" distance of L78.start L78.end
  measures "d91" distance of L82 L84
  measures "d92" distance of L81 L83
  measures "d93" distance of L67 L81
extrude "押し出し1'" add sketch "スケッチ1 (2)" against normal blind 2 separate body contours L40 L41 L42 L43 L44 A21 L45 L46 L47 A22 L48 L49 L50 L51 L52 L65 L66 L67 L68 L69 L70 L71 L72 L73 L74 L75 L76 L77 L81 L82 L83 L84 A26 A27 L85 L86 L87 A28 A29 | L79 L80 L84 makes body 11 in component "突起a"
sketch "スケッチ1 (3)" plane through (0, 0, 2) normal (0, 0, 1) x (-1, 0, 0) in component "突起b"
  circle A0 centre (-73.9241, 74.3082) radius 1.5
  circle A1 centre (101.3148, 26.8661) radius 1.5
  circle A2 centre (-27.3907, 101.1742) radius 1.5
  circle A3 centre (-26.8661, -101.3148) radius 1.5
  circle A4 centre (27.3907, 101.1742) radius 1.5
  circle A5 centre (101.3148, -26.8661) radius 1.5
  circle A6 centre (-101.3148, 26.8661) radius 1.5
  circle A7 centre (-101.3148, -26.8661) radius 1.5
  circle A8 centre (26.8661, -101.3148) radius 1.5
  circle A9 centre (73.9241, 74.3082) radius 1.5
  circle A10 centre (0, 0) radius 95
  line L0 (-71.3227, 78.5346) -> (-73.3227, 81.9987)
  arc A11 (-73.3227, 81.9987) -> (-107.6743, 22.5) centre (0, 0) ccw
  line L1 (-107.6743, 22.5) -> (-103.6743, 22.5)
  line L2 (-103.6743, 22.5) -> (-102.3148, 21.8661)
  line L3 (-102.3148, 21.8661) -> (-100.3148, 21.8661)
  line L4 (-100.3148, 21.8661) -> (-98.9554, 22.5)
  line L5 (-98.9554, 22.5) -> (-97.4359, 22.5)
  arc A12 (-97.4359, 22.5) -> (-99.6795, 8) centre (0, 0) ccw
  line L6 (-99.6795, 8) -> (-103.6795, 8)
  line L7 (-103.6795, 8) -> (-103.6795, -8)
  line L8 (-103.6795, -8) -> (-99.6795, -8)
  arc A13 (-99.6795, -8) -> (-97.4359, -22.5) centre (0, 0) ccw
  line L9 (-97.4359, -22.5) -> (-98.9554, -22.5)
  line L10 (-98.9554, -22.5) -> (-100.3148, -21.8661)
  line L11 (-100.3148, -21.8661) -> (-102.3148, -21.8661)
  line L12 (-102.3148, -21.8661) -> (-103.6743, -22.5)
  line L13 (-103.6743, -22.5) -> (-107.6743, -22.5)
  arc A14 (-107.6743, -22.5) -> (-22.5, -107.6743) centre (0, 0) ccw
  line L14 (-22.5, -107.6743) -> (-22.5, -103.6743)
  line L15 (-22.5, -103.6743) -> (-21.8661, -102.3148)
  line L16 (-21.8661, -102.3148) -> (-21.8661, -100.3148)
  line L17 (-21.8661, -100.3148) -> (-22.5, -98.9554)
  line L18 (-22.5, -98.9554) -> (-22.5, -97.4359)
  arc A15 (-22.5, -97.4359) -> (-8, -99.6795) centre (0, 0) ccw
  line L19 (-8, -99.6795) -> (-8, -103.6795)
  line L20 (-8, -103.6795) -> (8, -103.6795)
  line L21 (8, -103.6795) -> (8, -99.6795)
  arc A16 (8, -99.6795) -> (22.5, -97.4359) centre (0, 0) ccw
  line L22 (22.5, -97.4359) -> (22.5, -98.9554)
  line L23 (22.5, -98.9554) -> (21.8661, -100.3148)
  line L24 (21.8661, -100.3148) -> (21.8661, -102.3148)
  line L25 (21.8661, -102.3148) -> (22.5, -103.6743)
  line L26 (22.5, -103.6743) -> (22.5, -107.6743)
  arc A17 (22.5, -107.6743) -> (107.6743, -22.5) centre (0, 0) ccw
  line L27 (107.6743, -22.5) -> (103.6743, -22.5)
  line L28 (103.6743, -22.5) -> (102.3148, -21.8661)
  line L29 (102.3148, -21.8661) -> (100.3148, -21.8661)
  line L30 (100.3148, -21.8661) -> (98.9554, -22.5)
  line L31 (98.9554, -22.5) -> (97.4359, -22.5)
  arc A18 (97.4359, -22.5) -> (99.6795, -8) centre (0, 0) ccw
  line L32 (99.6795, -8) -> (103.6795, -8)
  line L33 (103.6795, -8) -> (103.6795, 8)
  line L34 (103.6795, 8) -> (99.6795, 8)
  arc A19 (99.6795, 8) -> (97.4359, 22.5) centre (0, 0) ccw
  line L35 (97.4359, 22.5) -> (98.9554, 22.5)
  line L36 (98.9554, 22.5) -> (100.3148, 21.8661)
  line L37 (100.3148, 21.8661) -> (102.3148, 21.8661)
  line L38 (102.3148, 21.8661) -> (103.6743, 22.5)
  line L39 (103.6743, 22.5) -> (107.6743, 22.5)
  arc A20 (107.6743, 22.5) -> (73.3227, 81.9987) centre (0, 0) ccw
  line L40 (73.3227, 81.9987) -> (71.3227, 78.5346)
  line L41 (71.3227, 78.5346) -> (70.094, 77.6742)
  line L42 (70.094, 77.6742) -> (69.094, 75.9421)
  line L43 (69.094, 75.9421) -> (68.9632, 74.4479)
  line L44 (68.9632, 74.4479) -> (68.2035, 73.1319)
  arc A21 (68.2035, 73.1319) -> (56.7679, 82.325) centre (0, 0) ccw
  line L45 (56.7679, 82.325) -> (58.7679, 85.7891)
  line L46 (58.7679, 85.7891) -> (44.9115, 93.7891)
  line L47 (44.9115, 93.7891) -> (42.9115, 90.325)
  arc A22 (42.9115, 90.325) -> (29.2324, 95.6319) centre (0, 0) ccw
  line L48 (29.2324, 95.6319) -> (29.9921, 96.9479)
  line L49 (29.9921, 96.9479) -> (31.2208, 97.8082)
  line L50 (31.2208, 97.8082) -> (32.2208, 99.5403)
  line L51 (32.2208, 99.5403) -> (32.3516, 101.0346)
  line L52 (32.3516, 101.0346) -> (34.3516, 104.4987)
  arc A23 (34.3516, 104.4987) -> (-34.3516, 104.4987) centre (0, 0) ccw
  line L53 (-34.3516, 104.4987) -> (-32.3516, 101.0346)
  line L54 (-32.3516, 101.0346) -> (-32.2208, 99.5403)
  line L55 (-32.2208, 99.5403) -> (-31.2208, 97.8082)
  line L56 (-31.2208, 97.8082) -> (-29.9921, 96.9479)
  line L57 (-29.9921, 96.9479) -> (-29.2324, 95.6319)
  arc A24 (-29.2324, 95.6319) -> (-42.9115, 90.325) centre (0, 0) ccw
  line L58 (-42.9115, 90.325) -> (-44.9115, 93.7891)
  line L59 (-44.9115, 93.7891) -> (-58.7679, 85.7891)
  line L60 (-58.7679, 85.7891) -> (-56.7679, 82.325)
  arc A25 (-56.7679, 82.325) -> (-68.2035, 73.1319) centre (0, 0) ccw
  line L61 (-68.2035, 73.1319) -> (-68.9632, 74.4479)
  line L62 (-68.9632, 74.4479) -> (-69.094, 75.9421)
  line L63 (-69.094, 75.9421) -> (-70.094, 77.6742)
  line L64 (-70.094, 77.6742) -> (-71.3227, 78.5346)
  line L65 (107.6743, -22.5) -> (103.6743, -22.5)
  line L66 (103.6743, -22.5) -> (102.3148, -21.8661)
  line L67 (102.3148, -21.8661) -> (100.3148, -21.8661)
  line L68 (100.3148, -21.8661) -> (98.9554, -22.5)
  line L69 (98.9554, -22.5) -> (97.4359, -22.5)
  line L70 (103.6795, -8) -> (99.6795, -8)
  line L71 (103.6795, -8) -> (103.6795, 0)
  line L72 (103.6795, 0) -> (163.6795, 0) construction
  line L73 (107.6743, -22.5) -> (163.6795, 0)
  line L74 (163.6795, 0) -> (107.6743, 22.5)
  line L75 (107.6743, -22.5) -> (107.6743, 22.5) construction
  line L76 (98.0068, -19.8661) -> (106.6743, -19.8661)
  line L77 (106.6743, -19.8661) -> (106.6743, -17.8661)
  line L78 (106.6743, -17.8661) -> (98.3911, -17.8661)
  arc A26 (97.4359, -22.5) -> (98.0068, -19.8661) centre (0, 0) ccw
  arc A27 (98.3911, -17.8661) -> (99.6795, -8) centre (0, 0) ccw
  line L79 (98.0068, 19.8661) -> (106.6743, 19.8661)
  line L80 (102.3148, 21.8661) -> (100.3148, 21.8661)
  line L81 (106.6743, 17.8661) -> (98.3911, 17.8661)
  arc A28 (99.6795, 8) -> (98.3911, 17.8661) centre (0, 0) ccw
  line L82 (103.6795, 8) -> (99.6795, 8)
  line L83 (103.6795, 8) -> (103.6795, 0)
  line L84 (106.6743, 19.8661) -> (106.6743, 17.8661)
  line L85 (100.3148, 21.8661) -> (98.9554, 22.5)
  line L86 (107.6743, 22.5) -> (103.6743, 22.5)
  line L87 (102.3148, 21.8661) -> (100.3148, 21.8661)
  line L88 (103.6743, 22.5) -> (102.3148, 21.8661)
  arc A29 (98.0068, 19.8661) -> (97.4359, 22.5) centre (0, 0) ccw
  line L89 (98.9554, 22.5) -> (97.4359, 22.5)
  line L90 (100.3148, 21.8661) -> (98.9554, 22.5)
  line L91 (107.6743, 22.5) -> (103.6743, 22.5)
  line L92 (98.9554, 22.5) -> (97.4359, 22.5)
  line L93 (99.6795, 8) -> (103.6795, 8)
  line L94 (103.6743, 22.5) -> (102.3148, 21.8661)
  arc A30 (99.6795, 8) -> (98.3911, 17.8661) centre (0, 0) ccw
  arc A31 (98.0068, 19.8661) -> (97.4359, 22.5) centre (0, 0) ccw
  point P0 (101.3148, 26.8661)
  point P1 (107.6743, 22.5)
  dimension "d96" = 60
  dimension "d97" = 1
  dimension "d98" = 2
  dimension "d99" = 2
  constraint coincident A17.end L27.start
  constraint coincident L27.end L28.start
  constraint coincident L28.end L29.start
  constraint coincident L29.end L30.start
  constraint coincident L30.end L31.start
  constraint coincident L31.end A18.start
  constraint coincident L32.end L33.start
  constraint coincident A18.end L32.start
  constraint midpoint L33 L71.end
  constraint coincident A10.centre A11.centre
  constraint perpendicular L33 L72
  constraint coincident P1 L39.end
  constraint horizontal L76
  constraint perpendicular L76 L77
  constraint coincident L78.end A26
  constraint perpendicular L77 L78
  constraint concentric A26 A27
  constraint symmetric A5.centre L72 P0
  constraint symmetric A17.end L72 P1
  constraint symmetric L27.end L72 L38.end
  constraint symmetric L28.end L72 L37.end
  constraint symmetric L29.end L72 L36.end
  constraint symmetric L30.end L72 L35.end
  constraint symmetric L31.end L72 A19.end
  constraint symmetric A18.end L72 L34.end
  constraint symmetric A18 L72 A30
  constraint symmetric L32.end L72 L33.end
  constraint symmetric L71.end L72 L83.end
  constraint symmetric L72 A17.end P1
  constraint symmetric L72 L76.start L79.start
  constraint symmetric L72 L76.end L79.end
  constraint symmetric L72 L77.end L81.start
  constraint symmetric L72 L78.end L81.end
  constraint symmetric L72 A26 A29
  constraint symmetric L72 A27 A28
  constraint concentric A30 A31
  measures "d96" distance of L71.end L72.end
  measures "d97" distance of L75 L77
  measures "d98" distance of L76 L78
  measures "d99" distance of L67 L76
extrude "押し出し1''" add sketch "スケッチ1 (3)" against normal blind 2 separate body contours L27 L28 L29 L30 L31 A18 L32 L33 L34 A19 L35 L36 L37 L38 L39 L65 L66 L67 L68 L69 L70 L71 L73 L74 L76 L77 L78 A26 A27 L79 L80 L81 A28 L82 L83 L84 L85 L86 L87 L88 A29 L89 L90 L91 L92 L93 L94 A30 A31 makes body 12 in component "突起b"
sketch "スケッチ1 (4)" plane through (0, 0, 2) normal (0, 0, 1) x (-1, 0, 0) in component "front"
  circle A0 centre (-73.9241, 74.3082) radius 1.5
  circle A1 centre (101.3148, 26.8661) radius 1.5
  circle A2 centre (-27.3907, 101.1742) radius 1.5
  circle A3 centre (-26.8661, -101.3148) radius 1.5
  circle A4 centre (27.3907, 101.1742) radius 1.5
  circle A5 centre (101.3148, -26.8661) radius 1.5
  circle A6 centre (-101.3148, 26.8661) radius 1.5
  circle A7 centre (-101.3148, -26.8661) radius 1.5
  circle A8 centre (26.8661, -101.3148) radius 1.5
  circle A9 centre (73.9241, 74.3082) radius 1.5
  circle A10 centre (0, 0) radius 95
  line L0 (-71.3227, 78.5346) -> (-73.3227, 81.9987)
  arc A11 (-73.3227, 81.9987) -> (-107.6743, 22.5) centre (0, 0) ccw
  line L1 (-107.6743, 22.5) -> (-103.6743, 22.5)
  line L2 (-103.6743, 22.5) -> (-102.3148, 21.8661)
  line L3 (-102.3148, 21.8661) -> (-100.3148, 21.8661)
  line L4 (-100.3148, 21.8661) -> (-98.9554, 22.5)
  line L5 (-98.9554, 22.5) -> (-97.4359, 22.5)
  arc A12 (-97.4359, 22.5) -> (-99.6795, 8) centre (0, 0) ccw
  line L6 (-99.6795, 8) -> (-103.6795, 8)
  line L7 (-103.6795, 8) -> (-103.6795, -8)
  line L8 (-103.6795, -8) -> (-99.6795, -8)
  arc A13 (-99.6795, -8) -> (-97.4359, -22.5) centre (0, 0) ccw
  line L9 (-97.4359, -22.5) -> (-98.9554, -22.5)
  line L10 (-98.9554, -22.5) -> (-100.3148, -21.8661)
  line L11 (-100.3148, -21.8661) -> (-102.3148, -21.8661)
  line L12 (-102.3148, -21.8661) -> (-103.6743, -22.5)
  line L13 (-103.6743, -22.5) -> (-107.6743, -22.5)
  arc A14 (-107.6743, -22.5) -> (-22.5, -107.6743) centre (0, 0) ccw
  line L14 (-22.5, -107.6743) -> (-22.5, -103.6743)
  line L15 (-22.5, -103.6743) -> (-21.8661, -102.3148)
  line L16 (-21.8661, -102.3148) -> (-21.8661, -100.3148)
  line L17 (-21.8661, -100.3148) -> (-22.5, -98.9554)
  line L18 (-22.5, -98.9554) -> (-22.5, -97.4359)
  arc A15 (-22.5, -97.4359) -> (-8, -99.6795) centre (0, 0) ccw
  line L19 (-8, -99.6795) -> (-8, -103.6795)
  line L20 (-8, -103.6795) -> (8, -103.6795)
  line L21 (8, -103.6795) -> (8, -99.6795)
  arc A16 (8, -99.6795) -> (22.5, -97.4359) centre (0, 0) ccw
  line L22 (22.5, -97.4359) -> (22.5, -98.9554)
  line L23 (22.5, -98.9554) -> (21.8661, -100.3148)
  line L24 (21.8661, -100.3148) -> (21.8661, -102.3148)
  line L25 (21.8661, -102.3148) -> (22.5, -103.6743)
  line L26 (22.5, -103.6743) -> (22.5, -107.6743)
  arc A17 (22.5, -107.6743) -> (107.6743, -22.5) centre (0, 0) ccw
  line L27 (107.6743, -22.5) -> (103.6743, -22.5)
  line L28 (103.6743, -22.5) -> (102.3148, -21.8661)
  line L29 (102.3148, -21.8661) -> (100.3148, -21.8661)
  line L30 (100.3148, -21.8661) -> (98.9554, -22.5)
  line L31 (98.9554, -22.5) -> (97.4359, -22.5)
  arc A18 (97.4359, -22.5) -> (99.6795, -8) centre (0, 0) ccw
  line L32 (99.6795, -8) -> (103.6795, -8)
  line L33 (103.6795, -8) -> (103.6795, 8)
  line L34 (103.6795, 8) -> (99.6795, 8)
  arc A19 (99.6795, 8) -> (97.4359, 22.5) centre (0, 0) ccw
  line L35 (97.4359, 22.5) -> (98.9554, 22.5)
  line L36 (98.9554, 22.5) -> (100.3148, 21.8661)
  line L37 (100.3148, 21.8661) -> (102.3148, 21.8661)
  line L38 (102.3148, 21.8661) -> (103.6743, 22.5)
  line L39 (103.6743, 22.5) -> (107.6743, 22.5)
  arc A20 (107.6743, 22.5) -> (73.3227, 81.9987) centre (0, 0) ccw
  line L40 (73.3227, 81.9987) -> (71.3227, 78.5346)
  line L41 (71.3227, 78.5346) -> (70.094, 77.6742)
  line L42 (70.094, 77.6742) -> (69.094, 75.9421)
  line L43 (69.094, 75.9421) -> (68.9632, 74.4479)
  line L44 (68.9632, 74.4479) -> (68.2035, 73.1319)
  arc A21 (68.2035, 73.1319) -> (56.7679, 82.325) centre (0, 0) ccw
  line L45 (56.7679, 82.325) -> (58.7679, 85.7891)
  line L46 (58.7679, 85.7891) -> (44.9115, 93.7891)
  line L47 (44.9115, 93.7891) -> (42.9115, 90.325)
  arc A22 (42.9115, 90.325) -> (29.2324, 95.6319) centre (0, 0) ccw
  line L48 (29.2324, 95.6319) -> (29.9921, 96.9479)
  line L49 (29.9921, 96.9479) -> (31.2208, 97.8082)
  line L50 (31.2208, 97.8082) -> (32.2208, 99.5403)
  line L51 (32.2208, 99.5403) -> (32.3516, 101.0346)
  line L52 (32.3516, 101.0346) -> (34.3516, 104.4987)
  arc A23 (34.3516, 104.4987) -> (-34.3516, 104.4987) centre (0, 0) ccw
  line L53 (-34.3516, 104.4987) -> (-32.3516, 101.0346)
  line L54 (-32.3516, 101.0346) -> (-32.2208, 99.5403)
  line L55 (-32.2208, 99.5403) -> (-31.2208, 97.8082)
  line L56 (-31.2208, 97.8082) -> (-29.9921, 96.9479)
  line L57 (-29.9921, 96.9479) -> (-29.2324, 95.6319)
  arc A24 (-29.2324, 95.6319) -> (-42.9115, 90.325) centre (0, 0) ccw
  line L58 (-42.9115, 90.325) -> (-44.9115, 93.7891)
  line L59 (-44.9115, 93.7891) -> (-58.7679, 85.7891)
  line L60 (-58.7679, 85.7891) -> (-56.7679, 82.325)
  arc A25 (-56.7679, 82.325) -> (-68.2035, 73.1319) centre (0, 0) ccw
  line L61 (-68.2035, 73.1319) -> (-68.9632, 74.4479)
  line L62 (-68.9632, 74.4479) -> (-69.094, 75.9421)
  line L63 (-69.094, 75.9421) -> (-70.094, 77.6742)
  line L64 (-70.094, 77.6742) -> (-71.3227, 78.5346)
  arc A26 (-29.3566, -90.3504) -> (0, -95) centre (0, 0) ccw
  line L65 (0, 0) -> (-29.3566, -90.3504) construction
  line L66 (0, 0) -> (0, -95) construction
  line L67 (-29.3566, -90.3504) -> (-33.9919, -104.6162)
  arc A27 (-33.9919, -104.6162) -> (0, -110) centre (0, 0) ccw
  line L68 (0, 0) -> (0, -110) construction
  circle A28 centre (-26.8661, -101.3148) radius 1.35
  arc A29 (0, -95) -> (29.3566, -90.3504) centre (0, 0) ccw
  line L69 (29.3566, -90.3504) -> (33.9919, -104.6162)
  circle A30 centre (26.8661, -101.3148) radius 1.35
  arc A31 (0, -110) -> (33.9919, -104.6162) centre (0, 0) ccw
  dimension "d102" = 18
  dimension "d104" = 15
  dimension "d106" = 2.7
  constraint coincident A10 A26.end
  constraint coincident A10.centre A11.centre
  constraint parallel L65 L67
  constraint concentric A3 A28
  constraint symmetric A26.start L66 A29.end
  constraint symmetric A26.end L66 A29.start
  constraint symmetric A26 L66 A29
  constraint symmetric L66 L67.end L69.end
  constraint symmetric L66 A27.end L68.end
  constraint symmetric L66 A27 A31
  constraint symmetric L66 A28 A30
  measures "d102" angle of L65 L66
  measures "d104" distance of A26.start L67.end
  measures "d106" diameter of A28
extrude "押し出し1'''" add sketch "スケッチ1 (4)" along normal blind 1 separate body contours A3 | A8 | A10 A14 L14 L15 L16 L17 L18 A15 L19 L20 L21 A16 L22 L23 L24 L25 L26 A17 A26 L67 A27 A29 L69 A31 | L14 L15 L16 L17 L18 A15 L19 L20 L21 A16 L22 L23 L24 L25 L26 A27 A31 | A28 | A30 makes body 13 in component "front"
extrude "押し出し2'" add sketch "スケッチ1 (4)" against normal blind 1 contours A28 | A30 bodies 13 in component "front"
copy_body "ボディのコピーと貼り付け1" bodies 13 makes body 14 in component "front"
move_body "移動1" bodies 14 to x (-1, 0, 0) y (0, 1, 0) z (0, 0, -1) at (-67.9837, 0, 2) in component "front"
move_body "移動2" bodies 14 to x (1, 0, 0) y (0, 1, 0) z (0, 0, 1) at (67.9837, 0, 0) in component "front"
copy_body "ボディ -> コンポーネント1" bodies 14 removing the originals makes body 15 in component "Component'''"
component "main" placed x (1, 0, 0) y (0, 1, 0) z (0, 0, 1) at (0, 0, 0)
component "突起a" placed x (1, 0, 0) y (0, 1, 0) z (0, 0, 1) at (0, 0, 0)
component "突起a" placed x (0.5, 0.866025, 0) y (-0.866025, 0.5, 0) z (0, 0, 1) at (0, 0, 0)
component "突起b" placed x (1, 0, 0) y (0, 1, 0) z (0, 0, 1) at (0, 0, 0)
component "突起b" placed x (0, -1, 0) y (1, 0, 0) z (0, 0, 1) at (0, 0, 0)
component "突起b" placed x (-1, 0, 0) y (0, -1, 0) z (0, 0, 1) at (0, 0, 0)
component "connector" placed x (1, 0, 0) y (0, 1, 0) z (0, 0, 1) at (0, 0, 0)
component "connector" placed x (0, -1, 0) y (1, 0, 0) z (0, 0, 1) at (0, 0, 0)
component "connector" placed x (-0.866025, -0.5, 0) y (0.5, -0.866025, 0) z (0, 0, 1) at (0, 0, 0)
component "connector" placed x (-0.866025, 0.5, 0) y (-0.5, -0.866025, 0) z (0, 0, 1) at (0, 0, 0)
component "connector" placed x (0, 1, 0) y (-1, 0, 0) z (0, 0, 1) at (0, 0, 0)
component "front" placed x (1, 0, 0) y (0, 1, 0) z (0, 0, 1) at (0, 0, 0) in component "connector"
component "Component'''" placed x (1, 0, 0) y (0, 1, 0) z (0, 0, 1) at (0, 0, 0) in component "front"
equation "d2 = d1 - 30 mm"
equation "d4 = d2 / 4"
equation "d5 = d4"
equation "d6 = d4"
equation "d8 = d4"
equation "d10 = d6"
equation "d11 = d3 + 10 mm"
equation "d13 = d12"
equation "d14 = d12"
equation "d15 = d12"
equation "d16 = d12"
equation "d17 = d12"
equation "d18 = d12"
equation "d19 = d12"
equation "d20 = d12"
equation "d21 = d12"
equation "d22 = ( d2 - 30 mm ) / 4"
equation "d23 = d22"
equation "d24 = d22"
equation "d26 = d25"
equation "d27 = d25"
equation "d29 = d28"
equation "d30 = d25 - 12 mm"
equation "d31 = d30"
equation "d32 = d30"
equation "d33 = d28 - 12 mm"
equation "d34 = d33"
equation "d35 = d30 / 3.5"
equation "d37 = d36"
equation "d38 = d35"
equation "d39 = d36"
equation "d40 = d36"
equation "d41 = d35"
equation "d42 = d36"
equation "d43 = d36"
equation "d44 = d33 / 4"
equation "d45 = d36"
equation "d46 = d36"
equation "d47 = d44"
equation "d48 = d36"
equation "d49 = d36"
equation "d69 = d54 / 2"
equation "d70 = d67"
equation "d71 = d68"
equation "d72 = d55 / 2"
equation "d78 = d75"
equation "d79 = d76"
